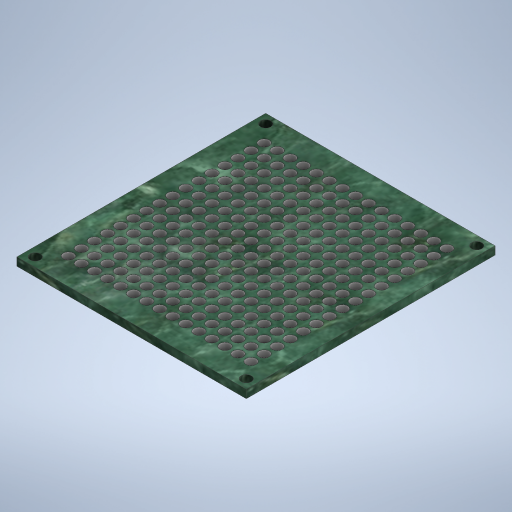
# Autodesk Inventor part: breadplate
Saved by Autodesk Inventor 2023 (Build 270158000, 158)
## iProperties
Created: 2023-09-25
Part Number: breadplate
Material: Generic
Document SubType Name: Modeling
Designer: Gage
Density: 1 g/cm^3
Appearance: Default
Author: Gage
Autodesk Inventor part; units mm, degrees
ref_plane "YZ Plane" through (0, 0, 0) normal (1, 0, 0) x (0, 1, 0)
ref_plane "XZ Plane" through (0, 0, 0) normal (0, 1, 0) x (-1, 0, 0)
ref_plane "XY Plane" through (0, 0, 0) normal (0, 0, 1) x (1, 0, 0)
sketch "Sketch1" plane through (0, 0, 0) normal (0, 1, 0) x (-1, 0, 0)
  line L0 (22.3242, -24.2094) -> (-22.3242, -24.2094)
  line L1 (-22.3242, -24.2094) -> (-22.3242, 24.2094)
  line L2 (-22.3242, 24.2094) -> (22.3242, 24.2094)
  line L3 (22.3242, 24.2094) -> (22.3242, -24.2094)
  point P0 (0, 0)
  point P1 (-22.3242, 0)
  point P2 (0, -24.2094)
  dimension "d0" = 44.6484
  dimension "d1" = 48.4188
  constraints: 8 end point, 2 midpoint, 2 parallel, 1 horizontal, 1 horizontal alignment, 1 perpendicular, 1 vertical alignment
  measures "d0" distance of L1.end L2.end
  measures "d1" distance of L0.end L1.end
extrude "Extrusion1" add sketch "Sketch1" along normal blind 1.5875
sketch "Sketch2" plane through (0, 1.5875, 0) normal (0, 1, 0) x (1, 0, 0)
  circle A0 centre (-20.5383, 22.4234) radius 0.9922
  line L0 (-22.3242, 24.2094) -> (-22.3242, -24.2094) projected
  line L1 (22.3242, 24.2094) -> (-22.3242, 24.2094) projected
  circle A1 centre (20.5383, 22.4234) radius 0.9922
  circle A2 centre (20.5383, -22.4234) radius 0.9922
  circle A3 centre (-20.5383, -22.4234) radius 0.9922
  line L2 (22.3242, -24.2094) -> (22.3242, 24.2094) projected
  line L3 (-22.3242, -24.2094) -> (22.3242, -24.2094) projected
  point P0 (0, 0)
  dimension "d4" = 1.9844
  dimension "d5" = 1.7859
  dimension "d6" = 1.7859
  dimension "d9" = 1.9844
  dimension "d10" = 1.9844
  dimension "d11" = 1.9844
  dimension "d12" = 1.7859
  dimension "d13" = 1.7859
  dimension "d14" = 1.7859
  dimension "d15" = 1.7859
  dimension "d16" = 1.7859
  dimension "d17" = 1.7859
  constraints: 4 centre point
  measures "d4" diameter of A0
  measures "d5" distance from line of L0 A0.centre
  measures "d6" distance from line of L1 A0.centre
  measures "d9" diameter of A1
  measures "d10" diameter of A2
  measures "d11" diameter of A3
  measures "d12" distance from line of L1 A1.centre
  measures "d13" distance from line of L2 A1.centre
  measures "d14" distance from line of L2 A2.centre
  measures "d15" distance from line of L3 A2.centre
  measures "d16" distance from line of L3 A3.centre
  measures "d17" distance from line of L0 A3.centre
extrude "Extrusion2" cut sketch "Sketch2" against normal blind 1.5875 contours A0 | A1 | A2 | A3
sketch "Sketch3" plane through (0, 1.5875, 0) normal (0, 1, 0) x (1, 0, 0)
  line L0 (-19.05, 20.6375) -> (19.05, 20.6375)
  line L1 (19.05, 20.6375) -> (19.05, -20.6375)
  line L2 (19.05, -20.6375) -> (-19.05, -20.6375)
  line L3 (-19.05, -20.6375) -> (-19.05, 20.6375)
  circle A0 centre (-17.4625, 19.05) radius 0.9922
  circle A1 centre (-17.4625, 16.51) radius 0.9922
  circle A2 centre (-17.4625, 13.97) radius 0.9922
  circle A3 centre (-17.4625, 11.43) radius 0.9922
  circle A4 centre (-17.4625, 8.89) radius 0.9922
  circle A5 centre (-17.4625, 6.35) radius 0.9922
  circle A6 centre (-17.4625, 3.81) radius 0.9922
  circle A7 centre (-17.4625, 1.27) radius 0.9922
  circle A8 centre (-17.4625, -1.27) radius 0.9922
  circle A9 centre (-17.4625, -3.81) radius 0.9922
  circle A10 centre (-17.4625, -6.35) radius 0.9922
  circle A11 centre (-17.4625, -8.89) radius 0.9922
  circle A12 centre (-17.4625, -11.43) radius 0.9922
  circle A13 centre (-17.4625, -13.97) radius 0.9922
  circle A14 centre (-17.4625, -16.51) radius 0.9922
  circle A15 centre (-17.4625, -19.05) radius 0.9922
  circle A16 centre (-14.9225, 19.05) radius 0.9922
  circle A17 centre (-14.9225, 16.51) radius 0.9922
  circle A18 centre (-14.9225, 13.97) radius 0.9922
  circle A19 centre (-14.9225, 11.43) radius 0.9922
  circle A20 centre (-14.9225, 8.89) radius 0.9922
  circle A21 centre (-14.9225, 6.35) radius 0.9922
  circle A22 centre (-14.9225, 3.81) radius 0.9922
  circle A23 centre (-14.9225, 1.27) radius 0.9922
  circle A24 centre (-14.9225, -1.27) radius 0.9922
  circle A25 centre (-14.9225, -3.81) radius 0.9922
  circle A26 centre (-14.9225, -6.35) radius 0.9922
  circle A27 centre (-14.9225, -8.89) radius 0.9922
  circle A28 centre (-14.9225, -11.43) radius 0.9922
  circle A29 centre (-14.9225, -13.97) radius 0.9922
  circle A30 centre (-14.9225, -16.51) radius 0.9922
  circle A31 centre (-14.9225, -19.05) radius 0.9922
  circle A32 centre (-12.3825, 19.05) radius 0.9922
  circle A33 centre (-12.3825, 16.51) radius 0.9922
  circle A34 centre (-12.3825, 13.97) radius 0.9922
  circle A35 centre (-12.3825, 11.43) radius 0.9922
  circle A36 centre (-12.3825, 8.89) radius 0.9922
  circle A37 centre (-12.3825, 6.35) radius 0.9922
  circle A38 centre (-12.3825, 3.81) radius 0.9922
  circle A39 centre (-12.3825, 1.27) radius 0.9922
  circle A40 centre (-12.3825, -1.27) radius 0.9922
  circle A41 centre (-12.3825, -3.81) radius 0.9922
  circle A42 centre (-12.3825, -6.35) radius 0.9922
  circle A43 centre (-12.3825, -8.89) radius 0.9922
  circle A44 centre (-12.3825, -11.43) radius 0.9922
  circle A45 centre (-12.3825, -13.97) radius 0.9922
  circle A46 centre (-12.3825, -16.51) radius 0.9922
  circle A47 centre (-12.3825, -19.05) radius 0.9922
  circle A48 centre (-9.8425, 19.05) radius 0.9922
  circle A49 centre (-9.8425, 16.51) radius 0.9922
  circle A50 centre (-9.8425, 13.97) radius 0.9922
  circle A51 centre (-9.8425, 11.43) radius 0.9922
  circle A52 centre (-9.8425, 8.89) radius 0.9922
  circle A53 centre (-9.8425, 6.35) radius 0.9922
  circle A54 centre (-9.8425, 3.81) radius 0.9922
  circle A55 centre (-9.8425, 1.27) radius 0.9922
  circle A56 centre (-9.8425, -1.27) radius 0.9922
  circle A57 centre (-9.8425, -3.81) radius 0.9922
  circle A58 centre (-9.8425, -6.35) radius 0.9922
  circle A59 centre (-9.8425, -8.89) radius 0.9922
  circle A60 centre (-9.8425, -11.43) radius 0.9922
  circle A61 centre (-9.8425, -13.97) radius 0.9922
  circle A62 centre (-9.8425, -16.51) radius 0.9922
  circle A63 centre (-9.8425, -19.05) radius 0.9922
  circle A64 centre (-7.3025, 19.05) radius 0.9922
  circle A65 centre (-7.3025, 16.51) radius 0.9922
  circle A66 centre (-7.3025, 13.97) radius 0.9922
  circle A67 centre (-7.3025, 11.43) radius 0.9922
  circle A68 centre (-7.3025, 8.89) radius 0.9922
  circle A69 centre (-7.3025, 6.35) radius 0.9922
  circle A70 centre (-7.3025, 3.81) radius 0.9922
  circle A71 centre (-7.3025, 1.27) radius 0.9922
  circle A72 centre (-7.3025, -1.27) radius 0.9922
  circle A73 centre (-7.3025, -3.81) radius 0.9922
  circle A74 centre (-7.3025, -6.35) radius 0.9922
  circle A75 centre (-7.3025, -8.89) radius 0.9922
  circle A76 centre (-7.3025, -11.43) radius 0.9922
  circle A77 centre (-7.3025, -13.97) radius 0.9922
  circle A78 centre (-7.3025, -16.51) radius 0.9922
  circle A79 centre (-7.3025, -19.05) radius 0.9922
  circle A80 centre (-4.7625, 19.05) radius 0.9922
  circle A81 centre (-4.7625, 16.51) radius 0.9922
  circle A82 centre (-4.7625, 13.97) radius 0.9922
  circle A83 centre (-4.7625, 11.43) radius 0.9922
  circle A84 centre (-4.7625, 8.89) radius 0.9922
  circle A85 centre (-4.7625, 6.35) radius 0.9922
  circle A86 centre (-4.7625, 3.81) radius 0.9922
  circle A87 centre (-4.7625, 1.27) radius 0.9922
  circle A88 centre (-4.7625, -1.27) radius 0.9922
  circle A89 centre (-4.7625, -3.81) radius 0.9922
  circle A90 centre (-4.7625, -6.35) radius 0.9922
  circle A91 centre (-4.7625, -8.89) radius 0.9922
  circle A92 centre (-4.7625, -11.43) radius 0.9922
  circle A93 centre (-4.7625, -13.97) radius 0.9922
  circle A94 centre (-4.7625, -16.51) radius 0.9922
  circle A95 centre (-4.7625, -19.05) radius 0.9922
  circle A96 centre (-2.2225, 19.05) radius 0.9922
  circle A97 centre (-2.2225, 16.51) radius 0.9922
  circle A98 centre (-2.2225, 13.97) radius 0.9922
  circle A99 centre (-2.2225, 11.43) radius 0.9922
  circle A100 centre (-2.2225, 8.89) radius 0.9922
  circle A101 centre (-2.2225, 6.35) radius 0.9922
  circle A102 centre (-2.2225, 3.81) radius 0.9922
  circle A103 centre (-2.2225, 1.27) radius 0.9922
  circle A104 centre (-2.2225, -1.27) radius 0.9922
  circle A105 centre (-2.2225, -3.81) radius 0.9922
  circle A106 centre (-2.2225, -6.35) radius 0.9922
  circle A107 centre (-2.2225, -8.89) radius 0.9922
  circle A108 centre (-2.2225, -11.43) radius 0.9922
  circle A109 centre (-2.2225, -13.97) radius 0.9922
  circle A110 centre (-2.2225, -16.51) radius 0.9922
  circle A111 centre (-2.2225, -19.05) radius 0.9922
  circle A112 centre (0.3175, 19.05) radius 0.9922
  circle A113 centre (0.3175, 16.51) radius 0.9922
  circle A114 centre (0.3175, 13.97) radius 0.9922
  circle A115 centre (0.3175, 11.43) radius 0.9922
  circle A116 centre (0.3175, 8.89) radius 0.9922
  circle A117 centre (0.3175, 6.35) radius 0.9922
  circle A118 centre (0.3175, 3.81) radius 0.9922
  circle A119 centre (0.3175, 1.27) radius 0.9922
  circle A120 centre (0.3175, -1.27) radius 0.9922
  circle A121 centre (0.3175, -3.81) radius 0.9922
  circle A122 centre (0.3175, -6.35) radius 0.9922
  circle A123 centre (0.3175, -8.89) radius 0.9922
  circle A124 centre (0.3175, -11.43) radius 0.9922
  circle A125 centre (0.3175, -13.97) radius 0.9922
  circle A126 centre (0.3175, -16.51) radius 0.9922
  circle A127 centre (0.3175, -19.05) radius 0.9922
  circle A128 centre (2.8575, 19.05) radius 0.9922
  circle A129 centre (2.8575, 16.51) radius 0.9922
  circle A130 centre (2.8575, 13.97) radius 0.9922
  circle A131 centre (2.8575, 11.43) radius 0.9922
  circle A132 centre (2.8575, 8.89) radius 0.9922
  circle A133 centre (2.8575, 6.35) radius 0.9922
  circle A134 centre (2.8575, 3.81) radius 0.9922
  circle A135 centre (2.8575, 1.27) radius 0.9922
  circle A136 centre (2.8575, -1.27) radius 0.9922
  circle A137 centre (2.8575, -3.81) radius 0.9922
  circle A138 centre (2.8575, -6.35) radius 0.9922
  circle A139 centre (2.8575, -8.89) radius 0.9922
  circle A140 centre (2.8575, -11.43) radius 0.9922
  circle A141 centre (2.8575, -13.97) radius 0.9922
  circle A142 centre (2.8575, -16.51) radius 0.9922
  circle A143 centre (2.8575, -19.05) radius 0.9922
  circle A144 centre (5.3975, 19.05) radius 0.9922
  circle A145 centre (5.3975, 16.51) radius 0.9922
  circle A146 centre (5.3975, 13.97) radius 0.9922
  circle A147 centre (5.3975, 11.43) radius 0.9922
  circle A148 centre (5.3975, 8.89) radius 0.9922
  circle A149 centre (5.3975, 6.35) radius 0.9922
  circle A150 centre (5.3975, 3.81) radius 0.9922
  circle A151 centre (5.3975, 1.27) radius 0.9922
  circle A152 centre (5.3975, -1.27) radius 0.9922
  circle A153 centre (5.3975, -3.81) radius 0.9922
  circle A154 centre (5.3975, -6.35) radius 0.9922
  circle A155 centre (5.3975, -8.89) radius 0.9922
  circle A156 centre (5.3975, -11.43) radius 0.9922
  circle A157 centre (5.3975, -13.97) radius 0.9922
  circle A158 centre (5.3975, -16.51) radius 0.9922
  circle A159 centre (5.3975, -19.05) radius 0.9922
  circle A160 centre (7.9375, 19.05) radius 0.9922
  circle A161 centre (7.9375, 16.51) radius 0.9922
  circle A162 centre (7.9375, 13.97) radius 0.9922
  circle A163 centre (7.9375, 11.43) radius 0.9922
  circle A164 centre (7.9375, 8.89) radius 0.9922
  circle A165 centre (7.9375, 6.35) radius 0.9922
  circle A166 centre (7.9375, 3.81) radius 0.9922
  circle A167 centre (7.9375, 1.27) radius 0.9922
  circle A168 centre (7.9375, -1.27) radius 0.9922
  circle A169 centre (7.9375, -3.81) radius 0.9922
  circle A170 centre (7.9375, -6.35) radius 0.9922
  circle A171 centre (7.9375, -8.89) radius 0.9922
  circle A172 centre (7.9375, -11.43) radius 0.9922
  circle A173 centre (7.9375, -13.97) radius 0.9922
  circle A174 centre (7.9375, -16.51) radius 0.9922
  circle A175 centre (7.9375, -19.05) radius 0.9922
  circle A176 centre (10.4775, 19.05) radius 0.9922
  circle A177 centre (10.4775, 16.51) radius 0.9922
  circle A178 centre (10.4775, 13.97) radius 0.9922
  circle A179 centre (10.4775, 11.43) radius 0.9922
  circle A180 centre (10.4775, 8.89) radius 0.9922
  circle A181 centre (10.4775, 6.35) radius 0.9922
  circle A182 centre (10.4775, 3.81) radius 0.9922
  circle A183 centre (10.4775, 1.27) radius 0.9922
  circle A184 centre (10.4775, -1.27) radius 0.9922
  circle A185 centre (10.4775, -3.81) radius 0.9922
  circle A186 centre (10.4775, -6.35) radius 0.9922
  circle A187 centre (10.4775, -8.89) radius 0.9922
  circle A188 centre (10.4775, -11.43) radius 0.9922
  circle A189 centre (10.4775, -13.97) radius 0.9922
  circle A190 centre (10.4775, -16.51) radius 0.9922
  circle A191 centre (10.4775, -19.05) radius 0.9922
  circle A192 centre (13.0175, 19.05) radius 0.9922
  circle A193 centre (13.0175, 16.51) radius 0.9922
  circle A194 centre (13.0175, 13.97) radius 0.9922
  circle A195 centre (13.0175, 11.43) radius 0.9922
  circle A196 centre (13.0175, 8.89) radius 0.9922
  circle A197 centre (13.0175, 6.35) radius 0.9922
  circle A198 centre (13.0175, 3.81) radius 0.9922
  circle A199 centre (13.0175, 1.27) radius 0.9922
  circle A200 centre (13.0175, -1.27) radius 0.9922
  circle A201 centre (13.0175, -3.81) radius 0.9922
  circle A202 centre (13.0175, -6.35) radius 0.9922
  circle A203 centre (13.0175, -8.89) radius 0.9922
  circle A204 centre (13.0175, -11.43) radius 0.9922
  circle A205 centre (13.0175, -13.97) radius 0.9922
  circle A206 centre (13.0175, -16.51) radius 0.9922
  circle A207 centre (13.0175, -19.05) radius 0.9922
  circle A208 centre (15.5575, 19.05) radius 0.9922
  circle A209 centre (15.5575, 16.51) radius 0.9922
  circle A210 centre (15.5575, 13.97) radius 0.9922
  circle A211 centre (15.5575, 11.43) radius 0.9922
  circle A212 centre (15.5575, 8.89) radius 0.9922
  circle A213 centre (15.5575, 6.35) radius 0.9922
  circle A214 centre (15.5575, 3.81) radius 0.9922
  circle A215 centre (15.5575, 1.27) radius 0.9922
  circle A216 centre (15.5575, -1.27) radius 0.9922
  circle A217 centre (15.5575, -3.81) radius 0.9922
  circle A218 centre (15.5575, -6.35) radius 0.9922
  circle A219 centre (15.5575, -8.89) radius 0.9922
  circle A220 centre (15.5575, -11.43) radius 0.9922
  circle A221 centre (15.5575, -13.97) radius 0.9922
  circle A222 centre (15.5575, -16.51) radius 0.9922
  circle A223 centre (15.5575, -19.05) radius 0.9922
  circle A224 centre (18.0975, 19.05) radius 0.9922
  circle A225 centre (18.0975, 16.51) radius 0.9922
  circle A226 centre (18.0975, 13.97) radius 0.9922
  circle A227 centre (18.0975, 11.43) radius 0.9922
  circle A228 centre (18.0975, 8.89) radius 0.9922
  circle A229 centre (18.0975, 6.35) radius 0.9922
  circle A230 centre (18.0975, 3.81) radius 0.9922
  circle A231 centre (18.0975, 1.27) radius 0.9922
  circle A232 centre (18.0975, -1.27) radius 0.9922
  circle A233 centre (18.0975, -3.81) radius 0.9922
  circle A234 centre (18.0975, -6.35) radius 0.9922
  circle A235 centre (18.0975, -8.89) radius 0.9922
  circle A236 centre (18.0975, -11.43) radius 0.9922
  circle A237 centre (18.0975, -13.97) radius 0.9922
  circle A238 centre (18.0975, -16.51) radius 0.9922
  circle A239 centre (18.0975, -19.05) radius 0.9922
  point P0 (0, 0)
  point P1 (19.05, -19.3278)
  point P2 (19.05, -18.7722)
  point P3 (19.05, -16.7878)
  point P4 (19.05, -16.2322)
  point P5 (19.05, 18.7722)
  point P6 (19.05, 19.3278)
  point P7 (19.05, 13.6922)
  point P8 (19.05, 14.2478)
  point P9 (19.05, 16.2322)
  point P10 (19.05, 16.7878)
  point P11 (19.05, 11.1522)
  point P12 (19.05, 11.7078)
  point P13 (19.05, 6.0722)
  point P14 (19.05, 6.6278)
  point P15 (19.05, 8.6122)
  point P16 (19.05, 9.1678)
  point P17 (19.05, 3.5322)
  point P18 (19.05, 4.0878)
  point P19 (19.05, 0.9922)
  point P20 (19.05, 1.5478)
  point P21 (19.05, -4.0878)
  point P22 (19.05, -3.5322)
  point P23 (19.05, -1.5478)
  point P24 (19.05, -0.9922)
  point P25 (19.05, -6.6278)
  point P26 (19.05, -6.0722)
  point P27 (19.05, -9.1678)
  point P28 (19.05, -8.6122)
  point P29 (19.05, -11.7078)
  point P30 (19.05, -11.1522)
  point P31 (19.05, -14.2478)
  point P32 (19.05, -13.6922)
  dimension "d18" = 1.9844
  dimension "d21" = 2.54
  dimension "d24" = 2.54
  constraints: 240 centre point, 15 equal radius, 15 vertical alignment, 6 end point, 3 horizontal, 1 parallel, 1 vertical, 451 other
  measures "d18" diameter of A0
  measures "d21" distance of A0.centre A1.centre
  measures "d24" distance of A0.centre A16.centre
extrude "Extrusion3" cut sketch "Sketch3" against normal blind 25.4 contours L1 A224 | A239 L1 | L1 A225 | A238 L1 | L1 A226 | A237 L1 | L1 A227 | A236 L1 | L1 A228 | A235 L1 | L1 A229 | A234 L1 | L1 A230 | A233 L1 | L1 A231 | A232 L1 | A0 | A1 | A2 | A3 | A4 | A5 | A6 | A7 | A8 | A9 | A10 | A11 | A12 | A13 | A14 | A15 | A16 | A17 | A18 | A19 | A20 | A21 | A22 | A23 | A24 | A25 | A26 | A27 | A28 | A29 | A30 | A31 | A32 | A33 | A34 | A35 | A36 | A37 | A38 | A39 | A40 | A41 | A42 | A43 | A44 | A45 | A46 | A47 | A48 | A49 | A50 | A51 | A52 | A53 | A54 | A55 | A56 | A57 | A58 | A59 | A60 | A61 | A62 | A63 | A64 | A65 | A66 | A67 | A68 | A69 | A70 | A71 | A72 | A73 | A74 | A75 | A76 | A77 | A78 | A79 | A80 | A81 | A82 | A83 | A84 | A85 | A86 | A87 | A88 | A89 | A90 | A91 | A92 | A93 | A94 | A95 | A96 | A97 | A98 | A99 | A100 | A101 | A102 | A103 | A104 | A105 | A106 | A107 | A108 | A109 | A110 | A111 | A112 | A113 | A114 | A115 | A116 | A117 | A118 | A119 | A120 | A121 | A122 | A123 | A124 | A125 | A126 | A127 | A128 | A129 | A130 | A131 | A132 | A133 | A134 | A135 | A136 | A137 | A138 | A139 | A140 | A141 | A142 | A143 | A144 | A145 | A146 | A147 | A148 | A149 | A150 | A151 | A152 | A153 | A154 | A155 | A156 | A157 | A158 | A159 | A160 | A161 | A162 | A163 | A164 | A165 | A166 | A167 | A168 | A169 | A170 | A171 | A172 | A173 | A174 | A175 | A176 | A177 | A178 | A179 | A180 | A181 | A182 | A183 | A184 | A185 | A186 | A187 | A188 | A189 | A190 | A191 | A192 | A193 | A194 | A195 | A196 | A197 | A198 | A199 | A200 | A201 | A202 | A203 | A204 | A205 | A206 | A207 | A208 | A209 | A210 | A211 | A212 | A213 | A214 | A215 | A216 | A217 | A218 | A219 | A220 | A221 | A222 | A223 picked at (18.2974, 19.3334) picked at (17.8937, -18.8251) picked at (18.3782, 16.8072) picked at (18.3919, -16.7057) picked at (18.2974, 14.2534) picked at (18.4043, -14.011) picked at (17.7543, 11.7157) picked at (18.4043, -11.389) picked at (18.1407, 8.5799) picked at (18.4043, -8.849) picked at (18.1407, 6.0399) picked at (18.4043, -6.309) picked at (18.2974, 4.0934) picked at (18.4043, -3.769) picked at (18.0599, 0.9461) picked at (18.4043, -1.311)
body "Solid1"
